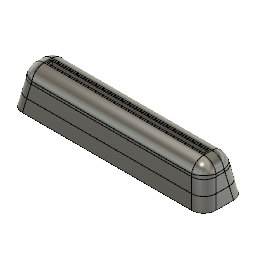
LEDStand_Final (Autodesk Fusion 360 design; units mm, degrees)
Autodesk Fusion 360 part; units mm, degrees
sketch "Sketch1" plane through (0, 0, 0) normal (0, 1, 0) x (1, 0, 0)
  line L0 (-72.6, 11.6) -> (72.6, 11.6)
  line L1 (72.6, 11.6) -> (72.6, -11.6)
  line L2 (72.6, -11.6) -> (-72.6, -11.6)
  line L3 (-72.6, -11.6) -> (-72.6, 11.6)
  line L4 (-72.6, 11.6) -> (72.6, -11.6) construction
  line L5 (72.6, 11.6) -> (-72.6, -11.6) construction
  dimension "d7" = 145.2
  dimension "d8" = 23.2
  constraint perpendicular L0 L1
  constraint parallel L0 L2
  constraint parallel L1 L3
  constraint horizontal L0
  constraint coincident L4 origin
  constraint coincident L5 origin
  measures "d7" distance of L0.start L0.end
  measures "d8" distance of L0.start L2.end
extrude "Extrude1" add sketch "Sketch1" along normal blind 30 makes body 1
sketch "Sketch2" plane through (0, 30, 0) normal (0, 1, 0) x (-1, 0, 0)
  line L0 (72.6, 11.6) -> (-72.6, 11.6)
  line L1 (-72.6, 11.6) -> (-72.6, -11.6)
  line L2 (-72.6, -11.6) -> (72.6, -11.6)
  line L3 (72.6, -11.6) -> (72.6, 11.6)
sketch "Sketch3" plane through (0, 30, 0) normal (0, 1, 0) x (-1, 0, 0)
  line L0 (-62.6, 1.6) -> (62.6, 1.6)
  line L1 (62.6, 1.6) -> (62.6, -1.6)
  line L2 (62.6, -1.6) -> (-62.6, -1.6)
  line L3 (-62.6, -1.6) -> (-62.6, 1.6)
  line L4 (-62.6, 1.6) -> (62.6, -1.6) construction
  line L5 (62.6, 1.6) -> (-62.6, -1.6) construction
  dimension "d11" = 3.2
  dimension "d12" = 125.2
  constraint perpendicular L0 L1
  constraint parallel L0 L2
  constraint parallel L1 L3
  constraint horizontal L0
  constraint coincident L4 origin
  constraint coincident L5 origin
  measures "d11" distance of L0.start L2.end
  measures "d12" distance of L0.start L0.end
extrude "Extrude2" cut sketch "Sketch3" against normal blind 10 bodies 1
ref_plane "WorkPlane3" through (0, 20, 0) normal (0, 1, 0) x (0, 0, 1)
ref_plane "WorkPlane4" through (0, 10, 0) normal (0, 1, 0) x (0, 0, 1)
draft "Draft1" angle 10 neutral plane through (0, 30, 0) pull (0, 1, 0) 2 faces at (24.2, 10, 11.6) (-24.2, 10, -11.6) on bodies 1
draft "Draft2" angle 10 neutral plane through (0, 30, 0) pull (0, 1, 0) 2 faces at (-72.6, 10, 3.8667) (72.6, 10, -3.8667) on bodies 1
fillet "Fillet3" radius 10 8 edges at (-75.2449, 15, 14.2449) (-75.2449, 15, -14.2449) (75.2449, 15, -14.2449) (75.2449, 15, 14.2449) (0, 30, 11.6) (72.6, 30, 0) (0, 30, -11.6) (-72.6, 30, 0) on bodies 1
chamfer "Chamfer2" distance 0.5 angle 45 4 edges at (0, 30, -1.6) (-62.6, 30, 0) (0, 30, 1.6) (62.6, 30, 0) on bodies 1
split "Split3" by plane through (0, 20, 0) normal (0, 1, 0) bodies 1 makes body 2 at (-21.403, 28.9363, -7.697)
split "Split4" by plane through (0, 10, 0) normal (0, 1, 0) bodies 1 makes body 3 at (20.8667, 20, -9.4422)
sketch "Sketch5" plane through (0, 10, 0) normal (0, 1, 0) x (-1, 0, 0)
  line L0 (76.1265, -5.2785) -> (76.1265, 5.2785)
  ellipse E0 centre (65.9723, 4.9723) end of major axis (73.2599, 12.2599) minor radius 10 (76.1265, 5.2785) -> (66.2785, 15.1265) ccw
  line L1 (66.2785, 15.1265) -> (-66.2785, 15.1265)
  ellipse E1 centre (-65.9723, 4.9723) end of major axis (-73.2599, 12.2599) minor radius 10 (-66.2785, 15.1265) -> (-76.1265, 5.2785) ccw
  line L2 (-76.1265, 5.2785) -> (-76.1265, -5.2785)
  ellipse E2 centre (-65.9723, -4.9723) end of major axis (-73.2599, -12.2599) minor radius 10 (-76.1265, -5.2785) -> (-66.2785, -15.1265) ccw
  line L3 (-66.2785, -15.1265) -> (66.2785, -15.1265)
  ellipse E3 centre (65.9723, -4.9723) end of major axis (73.2599, -12.2599) minor radius 10 (66.2785, -15.1265) -> (76.1265, -5.2785) ccw
  line L4 (70, -4.6) -> (-70, -4.6)
  line L5 (-70, -4.6) -> (-70, 4.6)
  line L6 (-70, 4.6) -> (70, 4.6)
  line L7 (70, 4.6) -> (70, -4.6)
  line L8 (70, -4.6) -> (-70, 4.6) construction
  line L9 (-70, -4.6) -> (70, 4.6) construction
  dimension "d30" = 9.2
  dimension "d31" = 140
  constraint perpendicular L4 L5
  constraint parallel L4 L6
  constraint parallel L5 L7
  constraint horizontal L4
  constraint coincident L8 origin
  constraint coincident L9 origin
  measures "d30" distance of L4.start L6.end
  measures "d31" distance of L4.start L4.end
extrude "Extrude10" cut sketch "Sketch5" along normal blind 10 contours L4 L5 L6 L7 bodies 3
extrude "Extrude3" cut sketch "Sketch5" along normal blind 10 contours L4 L5 L6 L7 bodies 3
sketch "Sketch7" plane through (0, 0, 0) normal (0, -1, 0) x (1, 0, 0)
  ellipse E0 centre (67.7355, -6.7355) end of major axis (75.0231, -14.0231) minor radius 10 (68.0417, -16.8898) -> (77.8898, -7.0417) ccw
  line L0 (77.8898, -7.0417) -> (77.8898, 7.0417)
  ellipse E1 centre (67.7355, 6.7355) end of major axis (75.0231, 14.0231) minor radius 10 (77.8898, 7.0417) -> (68.0417, 16.8898) ccw
  line L1 (68.0417, 16.8898) -> (-68.0417, 16.8898)
  ellipse E2 centre (-67.7355, 6.7355) end of major axis (-75.0231, 14.0231) minor radius 10 (-68.0417, 16.8898) -> (-77.8898, 7.0417) ccw
  line L2 (-77.8898, 7.0417) -> (-77.8898, -7.0417)
  ellipse E3 centre (-67.7355, -6.7355) end of major axis (-75.0231, -14.0231) minor radius 10 (-77.8898, -7.0417) -> (-68.0417, -16.8898) ccw
  line L3 (-68.0417, -16.8898) -> (68.0417, -16.8898)
  line L4 (-70, 10) -> (70, 10)
  line L5 (70, 10) -> (70, -10)
  line L6 (70, -10) -> (-70, -10)
  line L7 (-70, -10) -> (-70, 10)
  line L8 (-70, 10) -> (70, -10) construction
  line L9 (70, 10) -> (-70, -10) construction
  dimension "d38" = 140
  dimension "d39" = 20
  constraint perpendicular L4 L5
  constraint parallel L4 L6
  constraint parallel L5 L7
  constraint horizontal L4
  constraint coincident L8 origin
  constraint coincident L9 origin
  measures "d38" distance of L4.start L4.end
  measures "d39" distance of L4.start L6.end
extrude "Extrude5" cut sketch "Sketch7" against normal blind 4 contours L4 L5 L6 L7 bodies 1
sketch "Sketch11" plane through (0, 20, 0) normal (0, 1, 0) x (-1, 0, 0)
  line L0 (70, 4.6) -> (70, -4.6)
  line L1 (70, -4.6) -> (-70, -4.6)
  line L2 (-70, -4.6) -> (-70, 4.6)
  line L3 (-70, 4.6) -> (70, 4.6)
  ellipse E0 centre (64.209, 3.209) end of major axis (71.4966, 10.4966) minor radius 10 (74.3633, 3.5152) -> (64.5152, 13.3633) ccw
  line L4 (64.5152, 13.3633) -> (-64.5152, 13.3633)
  ellipse E1 centre (-64.209, 3.209) end of major axis (-71.4966, 10.4966) minor radius 10 (-64.5152, 13.3633) -> (-74.3633, 3.5152) ccw
  line L5 (-74.3633, 3.5152) -> (-74.3633, -3.5152)
  ellipse E2 centre (-64.209, -3.209) end of major axis (-71.4966, -10.4966) minor radius 10 (-74.3633, -3.5152) -> (-64.5152, -13.3633) ccw
  line L6 (-64.5152, -13.3633) -> (64.5152, -13.3633)
  ellipse E3 centre (64.209, -3.209) end of major axis (71.4966, -10.4966) minor radius 10 (64.5152, -13.3633) -> (74.3633, -3.5152) ccw
  line L7 (74.3633, -3.5152) -> (74.3633, 3.5152)
  line L8 (-70, 4.6) -> (-63, 4.6)
  line L9 (-63, 4.6) -> (-63, -15.4)
  line L10 (-63, -15.4) -> (-70, -15.4)
  line L11 (-70, -15.4) -> (-70, 4.6)
  dimension "d76" = 20
  dimension "d77" = 7
  constraint horizontal L8
  constraint vertical L9
  constraint horizontal L10
  constraint vertical L11
  constraint coincident L2.end L3.start
  measures "d76" distance of L2.end L10.end
  measures "d77" distance of L9.end L10.end
extrude "Extrude11" cut sketch "Sketch11" against normal blind 10 contours L1 L2 L3 L8 L9 L11 | L1 E2 L6 L9 L11 | E2 L6 L9 L10 L11 bodies 3
sketch "Sketch12" plane through (0, 10, 0) normal (0, 1, 0) x (-1, 0, 0)
  line L0 (76.1265, -5.2785) -> (76.1265, 5.2785)
  ellipse E0 centre (65.9723, 4.9723) end of major axis (73.2599, 12.2599) minor radius 10 (76.1265, 5.2785) -> (66.2785, 15.1265) ccw
  line L1 (66.2785, 15.1265) -> (-66.2785, 15.1265)
  ellipse E1 centre (-65.9723, 4.9723) end of major axis (-73.2599, 12.2599) minor radius 10 (-66.2785, 15.1265) -> (-76.1265, 5.2785) ccw
  line L2 (-76.1265, 5.2785) -> (-76.1265, -5.2785)
  ellipse E2 centre (-65.9723, -4.9723) end of major axis (-73.2599, -12.2599) minor radius 10 (-76.1265, -5.2785) -> (-66.2785, -15.1265) ccw
  line L3 (-66.2785, -15.1265) -> (66.2785, -15.1265)
  ellipse E3 centre (65.9723, -4.9723) end of major axis (73.2599, -12.2599) minor radius 10 (66.2785, -15.1265) -> (76.1265, -5.2785) ccw
  line L4 (68.3633, -8.3633) -> (-68.3633, -8.3633)
  line L5 (-68.3633, -8.3633) -> (-68.3633, 8.3633)
  line L6 (-68.3633, 8.3633) -> (68.3633, 8.3633)
  line L7 (68.3633, 8.3633) -> (68.3633, -8.3633)
  line L8 (68.3633, -8.3633) -> (-68.3633, 8.3633) construction
  line L9 (-68.3633, -8.3633) -> (68.3633, 8.3633) construction
  line L10 (74.3633, -3.5152) -> (74.3633, 3.5152)
  line L11 (-63, -13.3633) -> (64.5152, -13.3633)
  circle A0 centre (68.3633, -8.3633) radius 2.5
  circle A1 centre (68.3633, 8.3633) radius 2.5
  circle A2 centre (-68.3633, 8.3633) radius 2.5
  circle A3 centre (68.3633, -8.3633) radius 2.3
  circle A4 centre (68.3633, 8.3633) radius 2.3
  circle A5 centre (-68.3633, 8.3633) radius 2.3
  dimension "d80" = 6
  dimension "d81" = 5
  dimension "d82" = 5
  dimension "d83" = 5
  dimension "d84" = 5
  dimension "d87" = 0.2
  dimension "d88" = 0.2
  dimension "d89" = 0.2
  constraint perpendicular L4 L5
  constraint parallel L4 L6
  constraint parallel L5 L7
  constraint horizontal L4
  constraint coincident L8 origin
  constraint coincident L9 origin
  constraint coincident L4.start L7.end
  constraint coincident L6.end L7.start
  constraint coincident L5.end L6.start
  measures "d80" distance of L7 L10
  measures "d81" distance of L4 L11
  measures "d82" diameter of A0
  measures "d83" diameter of A1
  measures "d84" diameter of A2
extrude "Extrude13" add sketch "Sketch12" along normal blind 5 contours L4 L7 A3 | L4 L7 A3 | L6 L7 A4 | L6 L7 A4 | L5 L6 A5 | L5 L6 A5 bodies 1
extrude "Extrude12" cut sketch "Sketch12" along normal blind 4.8 contours L4 L7 A3 | L4 L7 A3 | L4 L7 A0 A3 | L4 L7 A0 A3 | L6 L7 A1 A4 | L6 L7 A1 A4 | L5 L6 A2 A5 | L5 L6 A2 A5 | L6 L7 A4 | L6 L7 A4 | L5 L6 A5 | L5 L6 A5 bodies 3
draft "Draft3" angle 5 neutral plane through (0, 10, 0) pull (0, 1, 0) 3 faces at (-67.4173, 11.6667, -6.2668) (-67.4173, 11.6667, 10.4597) (69.3092, 11.6667, 10.4597) on bodies 1
sketch "Sketch13" plane through (0, 20, 0) normal (0, 1, 0) x (-1, 0, 0)
  line L0 (-63, -4.6) -> (-63, -13.3633)
  line L1 (-63, -13.3633) -> (64.5152, -13.3633)
  ellipse E0 centre (64.209, -3.209) end of major axis (71.4966, -10.4966) minor radius 10 (64.5152, -13.3633) -> (74.3633, -3.5152) ccw
  line L2 (74.3633, -3.5152) -> (74.3633, 3.5152)
  ellipse E1 centre (64.209, 3.209) end of major axis (71.4966, 10.4966) minor radius 10 (74.3633, 3.5152) -> (64.5152, 13.3633) ccw
  line L3 (64.5152, 13.3633) -> (-64.5152, 13.3633)
  ellipse E2 centre (-64.209, 3.209) end of major axis (-71.4966, 10.4966) minor radius 10 (-64.5152, 13.3633) -> (-74.3633, 3.5152) ccw
  line L4 (-74.3633, 3.5152) -> (-74.3633, -3.5152)
  ellipse E3 centre (-64.209, -3.209) end of major axis (-71.4966, -10.4966) minor radius 10 (-74.3633, -3.5152) -> (-70, -11.7209) ccw
  line L5 (-70, -11.7209) -> (-70, 4.6)
  line L6 (-70, 4.6) -> (70, 4.6)
  line L7 (70, 4.6) -> (70, -4.6)
  line L8 (70, -4.6) -> (-63, -4.6)
  line L9 (66.5007, -8.3633) -> (-66.5007, -8.3633)
  line L10 (-66.5007, -8.3633) -> (-66.5007, 8.3633)
  line L11 (-66.5007, 8.3633) -> (66.5007, 8.3633)
  line L12 (66.5007, 8.3633) -> (66.5007, -8.3633)
  line L13 (66.5007, -8.3633) -> (-66.5007, 8.3633) construction
  line L14 (-66.5007, -8.3633) -> (66.5007, 8.3633) construction
  circle A0 centre (66.5007, -8.3633) radius 2.5
  circle A1 centre (66.5007, 8.3633) radius 2.5
  circle A2 centre (-66.5007, 8.3633) radius 2.5
  circle A3 centre (-66.5007, 8.3633) radius 2.3
  circle A4 centre (66.5007, -8.3633) radius 2.3
  circle A5 centre (66.5007, 8.3633) radius 2.3
  point P0 (66.5007, -8.3633)
  dimension "d94" = 5
  dimension "d95" = 5
  dimension "d96" = 5
  dimension "d97" = 0.2
  dimension "d98" = 0.2
  dimension "d99" = 0.2
  constraint perpendicular L9 L10
  constraint parallel L9 L11
  constraint parallel L10 L12
  constraint horizontal L9
  constraint coincident P0 L9.start
  constraint coincident L13 origin
  constraint coincident L14 origin
  constraint coincident L11.end L12.start
  constraint coincident L10.end L11.start
  measures "d94" diameter of A0
  measures "d95" diameter of A1
  measures "d96" diameter of A2
extrude "Extrude15" add sketch "Sketch13" along normal blind 4.8 contours L9 L12 A4 | L9 L12 A4 | L11 L12 A5 | L11 L12 A5 | L10 L11 A3 | L10 L11 A3 bodies 3
extrude "Extrude14" cut sketch "Sketch13" along normal blind 5 contours L9 L12 A0 A4 | L9 L12 A0 A4 | L9 L12 A4 | L9 L12 A4 | L11 L12 A1 A5 | L11 L12 A1 A5 | L10 L11 A2 A3 | L10 L11 A2 A3 | L11 L12 A5 | L11 L12 A5 | L10 L11 A3 | L10 L11 A3 bodies 2
draft "Draft4" angle 5 neutral plane through (0, 20, 0) pull (0, 1, 0) 1 faces at (-67.55, 21.6, 10.41) on bodies 3
draft "Draft5" angle 5 neutral plane through (0, 20, 0) pull (0, 1, 0) 1 faces at (-67.55, 21.6, -6.3166) on bodies 3
draft "Draft6" angle 5 neutral plane through (0, 20, 0) pull (0, 1, 0) 1 faces at (65.4514, 21.6, 10.41) on bodies 3
equation "OutsideLength = PaneLength + 20 mm"
equation "OutsideWidth = PaneWidth + 20 mm"
equation "PaneLength = 125.2 mm"
equation "PaneWidth = 3.2 mm"
equation "PaneDepth = 10 mm"
equation "OutsideHeight = 50 mm"
equation "d7 = OutsideLength"
equation "d8 = OutsideWidth"
equation "d11 = PaneWidth"
equation "d12 = PaneLength"
equation "d13 = -PaneDepth"
named bodies: "Bot (Dark)", "Bot (Dark) (1)", "Bot (Dark) (2)"
